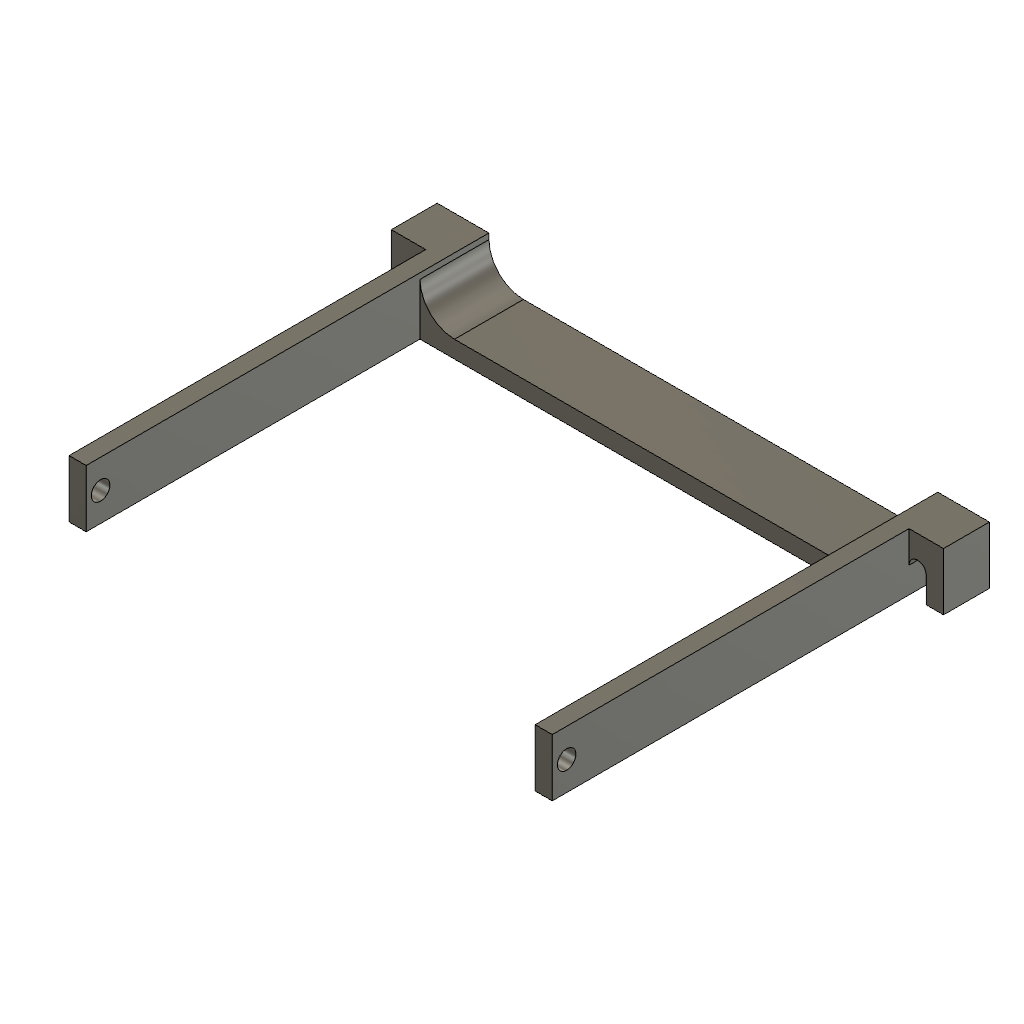
TankBot Phone Clamp (Autodesk Fusion 360 design; units mm, degrees)
Autodesk Fusion 360 part; units mm, degrees
box "BoxPrimitive1" add length 12 width 78 height 3 placed x (0, 0, 1) y (1, 0, 0) z (0, 1, 0) at (0, 0, 0)
box "BoxPrimitive2" add length 10 width 60 height 3 placed x (0, 1, 0) y (0, 0, 1) z (1, 0, 0) at (78, 0, 0)
box "BoxPrimitive3" add length 10 width 70 height 3 placed x (0, 1, 0) y (0, 0, -1) z (-1, 0, 0) at (0, 0, 70)
fillet "Fillet1" radius 6 1 edges at (78, 3, 6)
fillet "Fillet2" radius 6 1 edges at (0, 3, 6)
extrude "Extrude1" add 1 faces at (79, 6.6667, 60) along direction (0, 0, 1) blind 10
hole "Hole2" at (-3, 5, 67.5) direction (1, 0, 0) diameter 3.25 depth 160 tip angle 180
box "BoxPrimitive4" add length 4 width 8 height 3 placed x (0, -1, 0) y (0, 0, -1) z (1, 0, 0) at (81, 10, 8)
box "BoxPrimitive5" add length 4 width 8 height 3 placed x (0, -1, 0) y (0, 0, 1) z (-1, 0, 0) at (-3, 10, 0)
box "BoxPrimitive6" add length 10 width 8 height 3 placed x (0, -1, 0) y (0, 0, -1) z (1, 0, 0) at (84, 10, 8)
box "BoxPrimitive7" add length 10 width 8 height 3 placed x (0, -1, 0) y (0, 0, 1) z (-1, 0, 0) at (-6, 10, 0)
fillet "Fillet9" radius 1.5 1 edges at (84, 6, 4)
fillet "Fillet10" radius 1.5 1 edges at (81, 6, 4)
fillet "Fillet11" radius 1.5 1 edges at (-3, 6, 4)
fillet "Fillet12" radius 1.5 1 edges at (-6, 6, 4)
